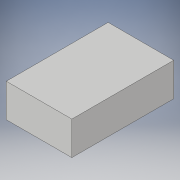
# Autodesk Inventor part: Part1
Saved by Autodesk Inventor 2018.2 (Build 222227000, 227)
## iProperties
Created: 2018-04-05
Part Number: Part1
Material: Generic
Document SubType Name: Modeling
Designer: Jose Munoz
Density: 1 g/cm^3
Appearance: Default
Author: Jose Munoz
Autodesk Inventor part; units mm, degrees
ref_plane "YZ Plane" through (0, 0, 0) normal (1, 0, 0) x (0, 1, 0)
ref_plane "XZ Plane" through (0, 0, 0) normal (0, 1, 0) x (-1, 0, 0)
ref_plane "XY Plane" through (0, 0, 0) normal (0, 0, 1) x (1, 0, 0)
sketch "Sketch1" plane through (0, 0, 0) normal (0, 0, 1) x (1, 0, 0)
  line L0 (-8.1723, 8.3142) -> (8.1723, 8.3142)
  line L1 (8.1723, 8.3142) -> (8.1723, 0)
  line L2 (8.1723, 0) -> (-8.1723, 0)
  line L3 (-8.1723, 0) -> (-8.1723, 8.3142)
  point P0 (0, 0)
  point P1 (0, 0)
  dimension "d0" = 16.3445
  dimension "d1" = 8.3142
  constraints: 8 end point, 2 coincident, 2 parallel, 1 horizontal, 1 midpoint, 1 perpendicular
  measures "d0" distance of L0.start L0.end
  measures "d1" distance of L2.end L0.start
extrude "Extrusion1" add sketch "Sketch1" along normal blind 25.4
body "Solid1"
